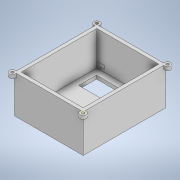
# Autodesk Inventor part: Spod
Saved by Autodesk Inventor 2021 (Build 250183000, 183)
## iProperties
Created: 2021-01-03
Part Number: Spod
Material: Generic
Document SubType Name: Modeling
Designer: emili
Density: 1 g/cm^3
Appearance: Default
Author: emili
Autodesk Inventor part; units mm, degrees
ref_plane "YZ Plane" through (0, 0, 0) normal (1, 0, 0) x (0, 1, 0)
ref_plane "XZ Plane" through (0, 0, 0) normal (0, 1, 0) x (-1, 0, 0)
ref_plane "XY Plane" through (0, 0, 0) normal (0, 0, 1) x (1, 0, 0)
sketch "Sketch2" plane through (0, 0, 0) normal (0, 1, 0) x (-1, 0, 0)
  line L0 (0, 0) -> (100, 0)
  line L1 (100, 0) -> (100, -120)
  line L2 (100, -120) -> (0, -120)
  line L3 (0, -120) -> (0, 0)
  dimension "d0" = 100
  dimension "d1" = 120
  constraints: 8 end point, 2 parallel, 1 horizontal, 1 perpendicular
  measures "d0" distance of L1.end L2.end
  measures "d1" distance of L0.end L1.end
extrude "Extrusion1" add sketch "Sketch2" along normal blind 5
sketch "Sketch3" plane through (0, 5, 0) normal (0, 1, 0) x (1, 0, 0)
  line L0 (0, 120) -> (-100, 120) projected
  line L1 (-100, 120) -> (-100, 0) projected
  line L2 (-95, 115) -> (-5, 115)
  line L3 (-5, 115) -> (-5, 5)
  line L4 (-5, 5) -> (-95, 5)
  line L5 (-95, 5) -> (-95, 115)
  line L6 (-100, 120) -> (0, 120)
  line L7 (0, 120) -> (0, 0)
  line L8 (0, 0) -> (-100, 0)
  line L9 (-100, 0) -> (-100, 120)
  dimension "d6" = 90
  dimension "d7" = 110
  constraints: 16 end point, 4 parallel, 2 horizontal, 2 perpendicular
  measures "d6" distance of L3.end L4.end
  measures "d7" distance of L2.end L3.end
extrude "Extrusion2" add sketch "Sketch3" along normal blind 50
sketch "Sketch5" plane through (0, 55, 0) normal (0, 1, 0) x (1, 0, 0)
  point P0 (0, 0)
sketch "Sketch6" plane through (0, 55, 0) normal (0, 1, 0) x (1, 0, 0)
  line L0 (-100, 0) -> (0, 0) projected
  line L1 (0, 0) -> (10, 0) construction
  circle A0 centre (1.4142, -1.4142) radius 2
  circle A1 centre (1.4142, -1.4142) radius 4.5
  circle A2 centre (1.4084, 121.4127) radius 2
  circle A3 centre (1.4084, 121.4127) radius 4.5
  circle A4 centre (-101.4585, 121.4298) radius 2
  circle A5 centre (-101.4585, 121.4298) radius 4.5
  circle A6 centre (-101.4195, -1.4184) radius 2
  circle A7 centre (-101.4195, -1.4184) radius 4.5
  dimension "d24" = 4
  dimension "d25" = 9
  dimension "d27" = 4
  dimension "d28" = 9
  dimension "d30" = 4
  dimension "d31" = 9
  dimension "d33" = 4
  dimension "d34" = 9
  constraints: 8 centre point, 4 coincident, 2 end point, 1 horizontal
  measures "d24" diameter of A0
  measures "d25" diameter of A1
  measures "d27" diameter of A2
  measures "d28" diameter of A3
  measures "d30" diameter of A4
  measures "d31" diameter of A5
  measures "d33" diameter of A6
  measures "d34" diameter of A7
extrude "Extrusion3" add sketch "Sketch6" against normal blind 5
sketch "Sketch7" plane through (0, 0, 0) normal (0, -1, 0) x (1, 0, 0)
  line L0 (-13.5, -106) -> (-86.5, -106)
  line L1 (-86.5, -106) -> (-86.5, -80)
  line L2 (-86.5, -80) -> (-13.5, -80)
  line L3 (-13.5, -80) -> (-13.5, -106)
  point P0 (0, 0)
  constraints: 8 end point, 2 parallel, 1 horizontal, 1 perpendicular
extrude "Extrusion4" cut sketch "Sketch7" against normal blind 10
sketch "Sketch8" plane through (0, 0, 0) normal (0, -1, 0) x (1, 0, 0)
  line L0 (-31, -62.5) -> (-69, -62.5)
  line L1 (-69, -62.5) -> (-69, -22.5)
  line L2 (-69, -22.5) -> (-31, -22.5)
  line L3 (-31, -22.5) -> (-31, -62.5)
  point P0 (0, 0)
  dimension "d48" = 38
  dimension "d49" = 40
  constraints: 8 end point, 2 parallel, 1 horizontal, 1 perpendicular
  measures "d48" distance of L1.end L2.end
  measures "d49" distance of L0.end L1.end
extrude "Extrusion5" cut sketch "Sketch8" against normal blind 10
sketch "Sketch9" plane through (0, 5, 0) normal (0, 1, 0) x (1, 0, 0)
  line L0 (-86.5, 106) -> (-13.5, 106) projected
  line L1 (-90, 106) -> (-90, 80)
  line L2 (-9.9472, 106) -> (-9.9472, 80)
  line L3 (-95, 115) -> (-95, 5) projected
  line L4 (-90, 106) -> (-95, 106)
  line L5 (-95, 106) -> (-95, 80)
  line L6 (-95, 80) -> (-90, 80)
  line L7 (-90, 80) -> (-90, 106)
  line L8 (-5, 5) -> (-5, 115) projected
  line L9 (-9.9472, 106) -> (-5, 106)
  line L10 (-5, 106) -> (-5, 80)
  line L11 (-5, 80) -> (-9.9472, 80)
  line L12 (-9.9472, 80) -> (-9.9472, 106)
  point P0 (0, 0)
  constraints: 20 end point, 4 parallel, 3 point on line, 2 horizontal, 2 perpendicular
extrude "Extrusion6" add sketch "Sketch9" along normal blind 9
sketch "Sketch10" plane through (-95, 5, -80) normal (0, 0, 1) x (1, 0, 0)
  line L0 (0, 0) -> (0, 9) projected
  line L1 (5, 0) -> (5, 9) projected
  line L2 (0, 9) -> (5, 9)
  line L3 (5, 9) -> (5, 0)
  line L4 (5, 0) -> (0, 0)
  line L5 (0, 0) -> (0, 9)
  point P0 (95, -5)
  constraints: 8 end point, 2 parallel, 1 horizontal, 1 perpendicular
extrude "Extrusion7" add sketch "Sketch10" along normal blind 5
sketch "Sketch11" plane through (-9.9472, 5, -80) normal (0, 0, 1) x (1, 0, 0)
  line L0 (4.9472, 0) -> (0, 0) projected
  line L1 (0, 9) -> (4.9472, 9)
  line L2 (4.9472, 9) -> (4.9472, 0)
  line L3 (4.9472, 0) -> (0, 0)
  line L4 (0, 0) -> (0, 9)
  point P0 (9.9472, -5)
  constraints: 8 end point, 2 parallel, 1 horizontal, 1 perpendicular
extrude "Extrusion8" add sketch "Sketch11" along normal blind 5
sketch "Sketch12" plane through (-5, 5, -106) normal (0, 0, -1) x (-1, 0, 0)
  line L0 (4.9472, 0) -> (4.9472, 9) projected
  line L1 (0, 9) -> (4.9472, 9)
  line L2 (4.9472, 9) -> (4.9472, 0)
  line L3 (4.9472, 0) -> (0, 0)
  line L4 (0, 0) -> (0, 9)
  line L5 (85, 0) -> (85, 9) projected
  line L6 (90, 0) -> (85, 0) projected
  line L7 (85, 9) -> (90, 9)
  line L8 (90, 9) -> (90, 0)
  line L9 (90, 0) -> (85, 0)
  line L10 (85, 0) -> (85, 9)
  point P0 (-5, -5)
  constraints: 16 end point, 4 parallel, 2 horizontal, 2 perpendicular
extrude "Extrusion9" add sketch "Sketch12" along normal blind 10
sketch "Sketch13" plane through (-9.9472, 5, -115) normal (-1, 0, 0) x (0, 0, 1)
  line L0 (0, 0) -> (0, 9) projected
  line L1 (40, 9) -> (40, 0) projected
  line L2 (0, 9) -> (40, 9)
  line L3 (40, 9) -> (40, 4)
  line L4 (40, 4) -> (0, 4)
  line L5 (0, 4) -> (0, 9)
  point P0 (115, -5)
  dimension "d62" = 5
  constraints: 8 end point, 2 parallel, 1 horizontal, 1 perpendicular, 1 point on line
  measures "d62" distance of L2.end L3.end
extrude "Extrusion10" add sketch "Sketch13" along normal blind 6
sketch "Sketch14" plane through (-90, 5, -115) normal (1, 0, 0) x (0, 0, -1)
  line L0 (0, 9) -> (0, 0) projected
  line L1 (0, 9) -> (-39.9886, 9)
  line L2 (-39.9886, 9) -> (-39.9886, 4)
  line L3 (-39.9886, 4) -> (0, 4)
  line L4 (0, 4) -> (0, 9)
  point P0 (-115, -5)
  dimension "d65" = 5
  constraints: 8 end point, 2 parallel, 1 horizontal, 1 perpendicular
  measures "d65" distance of L2.end L1.end
extrude "Extrusion11" add sketch "Sketch14" along normal blind 6
sketch "Sketch15" plane through (-69, 0, -62.5) normal (0, 0, 1) x (1, 0, 0)
  line L0 (0, 5) -> (38, 5) projected
  line L1 (38, 0) -> (38, 5) projected
  line L2 (0, 5) -> (38, 5)
  line L3 (38, 5) -> (38, 0)
  line L4 (38, 0) -> (0, 0)
  line L5 (0, 0) -> (0, 5)
  point P0 (69, 0)
  constraints: 8 end point, 2 parallel, 1 horizontal, 1 perpendicular
extrude "Extrusion12" add sketch "Sketch15" along normal blind 10
sketch "Sketch16" plane through (-31, 0, -22.5) normal (0, 0, -1) x (-1, 0, 0)
  line L0 (0, 5) -> (38, 5) projected
  line L1 (38, 0) -> (0, 0) projected
  line L2 (0, 5) -> (38, 5)
  line L3 (38, 5) -> (38, 0)
  line L4 (38, 0) -> (0, 0)
  line L5 (0, 0) -> (0, 5)
  point P0 (-31, 0)
  constraints: 8 end point, 2 parallel, 1 horizontal, 1 perpendicular
extrude "Extrusion13" cut sketch "Sketch16" against normal blind 10
sketch "Sketch17" plane through (-9.9472, 5, -75) normal (0, 0, 1) x (1, 0, 0)
  line L0 (4.9472, 9) -> (-6, 9) projected
  line L1 (4.9472, 9) -> (-6, 9)
  line L2 (-6, 4) -> (-6, 9) projected
  line L3 (-6, 9) -> (-6, 4)
  line L4 (0, 4) -> (0, 0) projected
  line L5 (-6, 4) -> (0, 4)
  line L6 (0, 4) -> (0, 0)
  line L7 (4.9472, 9) -> (4.9472, 0) projected
  line L8 (0, 0) -> (4.9472, 0)
  line L9 (4.9472, 0) -> (4.9472, 9)
  point P0 (9.9472, -5)
  constraints: 12 end point, 5 perpendicular, 1 horizontal
extrude "Extrusion14" cut sketch "Sketch17" against normal blind 40
sketch "Sketch18" plane through (-90, 9, -75.0114) normal (0, 0, 1) x (1, 0, 0)
  line L0 (0, 5) -> (6, 5) projected
  line L1 (-5, -4) -> (-5, 5) projected
  line L2 (6, 5) -> (-5, 5)
  line L3 (-5, 5) -> (-5, -4)
  line L4 (0, -4) -> (-5, -4) projected
  line L5 (-5, -4) -> (0, -4)
  line L6 (0, -4) -> (0, 0)
  line L7 (0, -4) -> (0, 5) projected
  line L8 (6, 5) -> (6, 0) projected
  line L9 (6, 5) -> (6, 0)
  point P0 (90, -9)
  dimension "d74" = 4
  constraints: 10 end point, 3 collinear, 1 horizontal, 1 point on line
  measures "d74" distance of L4.start L6.end
extrude "Extrusion15" cut sketch "Sketch18" against normal blind 40
sketch "Sketch19" plane through (-84, 9, -75.0114) normal (0, 0, 1) x (1, 0, 0)
  line L0 (0, 5) -> (0, 0) projected
  line L1 (0, 0) -> (0, 5)
  line L2 (0, 5) -> (-6, 5)
  line L3 (-6, 0) -> (0, 0) projected
  line L4 (-6, 5) -> (-6, 0)
  line L5 (-6, 0) -> (0, 0)
  point P0 (84, -9)
  constraints: 8 end point, 2 perpendicular, 1 collinear, 1 vertical
extrude "Extrusion16" cut sketch "Sketch19" against normal blind 40
sketch "Sketch20" plane through (-95, 5, -75) normal (0, 0, 1) x (1, 0, 0)
  line L0 (0, 9) -> (0, 0) projected
  line L1 (5, 9) -> (0, 9)
  line L2 (0, 9) -> (0, 0)
  line L3 (0, 0) -> (5, 0)
  line L4 (5, 0) -> (5, 9)
  point P0 (95, -5)
  constraints: 8 end point, 2 parallel, 1 horizontal, 1 perpendicular
extrude "Extrusion17" cut sketch "Sketch20" against normal blind 10
body "Solid1"
